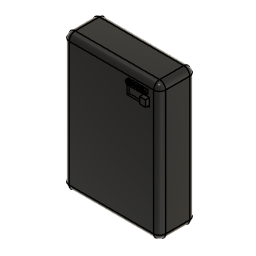
Caja+Pilas (Autodesk Fusion 360 design; units mm, degrees)
Autodesk Fusion 360 part; units mm, degrees
sketch "Sketch1" plane through (0, 0, 0) normal (0, 1, 0) x (1, 0, 0)
  line L0 (0, 0) -> (48, 0)
  line L1 (48, 0) -> (48, -68)
  line L2 (48, -68) -> (0, -68)
  line L3 (0, -68) -> (0, 0)
  dimension "d1" = 48
  dimension "d2" = 68
  constraint horizontal L0
  constraint vertical L1
  constraint horizontal L2
  constraint vertical L3
  constraint coincident L0.start L3.end
  measures "d1" distance of L0.start L0.end
  measures "d2" distance of L0.start L2.end
extrude "Extrude1" add sketch "Sketch1" along normal blind 18
fillet "Fillet1" radius 3 12 edges at (48, 9, 68) (24, 18, 68) (24, 0, 68) (48, 0, 34) (48, 9, 0) (24, 18, 0) (24, 0, 0) (0, 9, 0) (0, 0, 34) (0, 18, 34) (0, 9, 68) (48, 18, 34)
sketch "Boceto2" plane through (0, 0, 0) normal (0, -1, 0) x (1, 0, 0)
  line L0 (45, 65) -> (3, 65)
  line L1 (3, 65) -> (3, 3)
  line L2 (3, 3) -> (45, 3)
  line L3 (45, 3) -> (45, 65)
  line L4 (31.7729, 60.7203) -> (42.8614, 60.7203)
  line L5 (42.8614, 60.7203) -> (42.8614, 56.4555)
  line L6 (42.8614, 56.4555) -> (31.7729, 56.4555)
  line L7 (31.7729, 56.4555) -> (31.7729, 60.7203)
  constraint horizontal L4
  constraint vertical L5
  constraint horizontal L6
  constraint vertical L7
extrude "Extruir2" cut sketch "Boceto2" against normal blind 1 contours L4 L5 L6 L7
sketch "Boceto3" plane through (0, 1, 0) normal (0, -1, 0) x (1, 0, 0)
  line L0 (31.7729, 56.4555) -> (42.8614, 56.4555)
  line L1 (42.8614, 56.4555) -> (42.8614, 60.7203)
  line L2 (42.8614, 60.7203) -> (31.7729, 60.7203)
  line L3 (31.7729, 60.7203) -> (31.7729, 56.4555)
  line L4 (39.5545, 60.2451) -> (42.5, 60.2451)
  line L5 (42.5, 60.2451) -> (42.5, 57)
  line L6 (42.5, 57) -> (39.5545, 57)
  line L7 (39.5545, 57) -> (39.5545, 60.2451)
  constraint horizontal L4
  constraint vertical L5
  constraint horizontal L6
  constraint vertical L7
extrude "Extruir3" add sketch "Boceto3" along normal blind 2.5 contours L4 L5 L6 L7
sketch "Boceto4" plane through (0, 0, 0) normal (0, -1, 0) x (1, 0, 0)
  line L0 (42.8614, 60.7203) -> (42.8614, 56.4555)
  line L1 (42.8614, 56.4555) -> (31.7729, 56.4555)
  line L2 (31.7729, 56.4555) -> (31.7729, 60.7203)
  line L3 (31.7729, 60.7203) -> (42.8614, 60.7203)
  line L4 (45, 65) -> (3, 65)
  line L5 (3, 65) -> (3, 3)
  line L6 (3, 3) -> (45, 3)
  line L7 (45, 3) -> (45, 65)
  line L8 (31.9974, 60.7278) -> (41.3548, 60.7203) construction
  line L9 (41.3548, 60.7203) -> (41.3575, 63.9925) construction
  line L10 (41.3575, 63.9925) -> (32, 64) construction
  line L11 (32, 64) -> (31.9974, 60.7278) construction
  dimension "d11" = 2
  text T0 "OFF/ON" font "Arial" height 2 align left top in box 9.3575 x 3.2722 at (31.9974, 60.7278) x (1, -0.000799) y (0.000799, 1) spacing 1
  constraint coincident L3
extrude "Extruir4" add sketch "Boceto4" along normal blind 1 text T0
